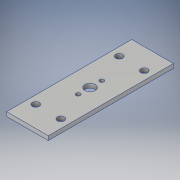
# Autodesk Inventor part: 板 中心Φ7
Saved by Autodesk Inventor 2019 (Build 230136000, 136)
## iProperties
Created: 2020-10-08
Part Number: 板 中心Φ7
Material: アルミニウム 6061
Document SubType Name: Modeling
Designer: zhept
Density: 2.7 g/cm^3
Appearance: アルミニウム - フラット
Author: zhept
Autodesk Inventor part; units mm, degrees
ref_plane "YZ Plane" through (0, 0, 0) normal (1, 0, 0) x (0, 1, 0)
ref_plane "XZ Plane" through (0, 0, 0) normal (0, 1, 0) x (-1, 0, 0)
ref_plane "XY Plane" through (0, 0, 0) normal (0, 0, 1) x (1, 0, 0)
sketch "スケッチ1" plane through (0, 0, 0) normal (0, 1, 0) x (-1, 0, 0)
  circle A0 centre (0, 0) radius 12.5
  line L0 (-15, -45) -> (-15, 45)
  line L1 (-15, 45) -> (15, 45)
  line L2 (15, 45) -> (15, -45)
  line L3 (15, -45) -> (-15, -45)
  line L4 (-15, -45) -> (15, 45) construction
  line L5 (-15, 45) -> (15, -45) construction
  circle A1 centre (0, -8.5) radius 1.5
  circle A2 centre (0, 8.5) radius 1.5
  dimension "d0" = 25
  dimension "d1" = 90
  dimension "d2" = 30
  dimension "d10" = 3
  dimension "d11" = 3
  constraints: 12 end point, 3 centre point, 2 midpoint, 2 parallel, 1 coincident, 1 perpendicular, 1 vertical
  measures "d0" diameter of A0
  measures "d1" distance of L0.start L0.end
  measures "d2" distance of L0.end L1.end
  measures "d10" diameter of A1
  measures "d11" diameter of A2
extrude "押し出し3" add sketch "スケッチ1" along normal blind 3 contours A0 | L0 L1 L2 L3
sketch "スケッチ3" plane through (0, 3, 0) normal (0, 1, 0) x (1, 0, 0)
  circle A0 centre (0, 0) radius 3.75
  dimension "d14" = 7.5
  constraints: 1 centre point, 1 coincident
  measures "d14" diameter of A0
extrude "押し出し4" cut sketch "スケッチ3" against normal blind 3
sketch "スケッチ4" plane through (0, 3, 0) normal (0, 1, 0) x (1, 0, 0)
  line L0 (0, 0) -> (0, 30)
  line L1 (0, 30) -> (0, -30)
  line L2 (0, -30) -> (-9, -30)
  line L3 (-15, 45) -> (-15, -45) projected
  circle A0 centre (-9, -30) radius 2.5
  line L4 (0, -30) -> (9, -30)
  line L5 (9, -30) -> (-9, 30)
  line L6 (-9, -30) -> (9, 30)
  circle A1 centre (9, -30) radius 2.5
  circle A2 centre (-9, 30) radius 2.5
  circle A3 centre (9, 30) radius 2.5
  dimension "d17" = 30
  dimension "d18" = 60
  dimension "d19" = 9
  dimension "d20" = 5
  dimension "d21" = 9
  dimension "d23" = 5
  dimension "d24" = 5
  dimension "d25" = 5
  constraints: 12 end point, 4 centre point, 4 coincident, 1 horizontal, 1 perpendicular, 1 point on line, 1 vertical
  measures "d17" distance of L0.start L0.end
  measures "d18" distance of L0.end L1.end
  measures "d19" distance of L1.end L2.end
  measures "d20" diameter of A0
  measures "d21" distance of L1.end L4.end
  measures "d23" diameter of A1
  measures "d24" diameter of A2
  measures "d25" diameter of A3
extrude "押し出し5" cut sketch "スケッチ4" against normal blind 3 contours A2 | A3 | A1 L4 L5 | L5 L4 A1 | L6 L2 A0 | A0 L2 L6
